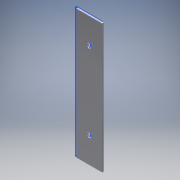
# Autodesk Inventor part: basicLiftPlate
Saved by Autodesk Inventor 2016 SP1 (Build 200210100, 210)
## iProperties
Created: 2016-02-01
Part Number: basicLiftPlate
Material: Aluminum 6061
Document SubType Name: Modeling
Designer: steele
Density: 2.7 g/cm^3
Appearance: Aluminum - Flat
Mass: 109.391 g
Surface Area: 276.469 cm^2
Volume: 40.5152 cm^3
Author: steele
Autodesk Inventor part; units mm, degrees
ref_plane "YZ Plane" through (0, 0, 0) normal (1, 0, 0) x (0, 1, 0)
ref_plane "XZ Plane" through (0, 0, 0) normal (0, 1, 0) x (-1, 0, 0)
ref_plane "XY Plane" through (0, 0, 0) normal (0, 0, 1) x (1, 0, 0)
sketch "Sketch1" plane through (0, 0, 0) normal (0, 0, 1) x (1, 0, 0)
  line L0 (-25.4, -127) -> (25.4, -127)
  line L1 (25.4, -127) -> (25.4, 127)
  line L2 (25.4, 127) -> (-25.4, 127)
  line L3 (-25.4, 127) -> (-25.4, -127)
  line L4 (-25.4, -127) -> (25.4, 127) construction
  line L5 (25.4, -127) -> (-25.4, 127) construction
  point P0 (0, 0)
  dimension "d0" = 50.8
  dimension "d1" = 254
  constraints: 12 end point, 2 midpoint, 2 parallel, 1 horizontal, 1 perpendicular
  measures "d0" distance of L0.start L0.end
  measures "d1" distance of L2.end L0.start
extrude "Extrusion1" add sketch "Sketch1" along normal blind 3.175
sketch "Sketch2" plane through (0, 0, 3.175) normal (0, 0, 1) x (1, 0, 0)
  line L0 (25.4, 127) -> (-25.4, 127) construction
  line L1 (0, 127) -> (0, -127) construction
  line L2 (-25.4, -127) -> (25.4, -127) construction
  circle A0 centre (0, 76.2) radius 4.7625
  circle A1 centre (0, -76.2) radius 4.7625
  point P0 (0, 0)
  dimension "d4" = 50.8
  dimension "d5" = 50.8
  dimension "d6" = 9.525
  dimension "d7" = 9.525
  constraints: 2 centre point, 2 end point, 2 midpoint, 2 point on line
  measures "d4" distance from line of A0.centre L0
  measures "d5" distance of A1.centre L1.end
  measures "d6" diameter of A1
  measures "d7" diameter of A0
extrude "Extrusion2" cut sketch "Sketch2" against normal through all
equation "\"d0\" = basicLiftWidth"
equation "\"d1\" = basicLiftLength"
equation "\"d2\" = basicLiftThickness"
equation "\"d4\" = basicLLiftAxelsDistanceFromTop"
equation "\"d5\" = basicLiftaxelDistancefromBottom"
equation "\"d6\" = baslicLiftAxelDiam"
equation "\"d7\" = baslicLiftAxelDiam"
equation "\"basicLiftLength\" = 254"
equation "\"basicLiftWidth\" = 50.8"
equation "\"basicLiftaxelDistancefromBottom\" = 50.8"
equation "\"basicLLiftAxelsDistanceFromTop\" = 50.8"
equation "\"basicLiftThickness\" = 3.175"
equation "\"baslicLiftAxelDiam\" = 9.525"
body "Solid1"
